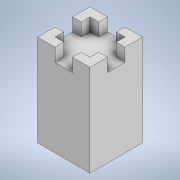
# Autodesk Inventor part: rook
Saved by Autodesk Inventor 2021 (Build 250183000, 183)
## iProperties
Created: 2021-01-20
Part Number: rook
Material: Generic
Document SubType Name: Modeling
Designer: Luke Kamols
Density: 1 g/cm^3
Appearance: Default
Author: Luke Kamols
Autodesk Inventor part; units mm, degrees
ref_plane "YZ Plane" through (0, 0, 0) normal (1, 0, 0) x (0, 1, 0)
ref_plane "XZ Plane" through (0, 0, 0) normal (0, 1, 0) x (-1, 0, 0)
ref_plane "XY Plane" through (0, 0, 0) normal (0, 0, 1) x (1, 0, 0)
sketch "Sketch1" plane through (0, 0, 0) normal (0, 1, 0) x (-1, 0, 0)
  line L0 (0, 0) -> (20, 0)
  line L1 (20, 0) -> (20, -20)
  line L2 (20, -20) -> (0, -20)
  line L3 (0, -20) -> (0, 0)
  dimension "d0" = 20
  dimension "d1" = 20
  constraints: 8 end point, 2 parallel, 1 horizontal, 1 perpendicular
  measures "d0" distance of L1.end L2.end
  measures "d1" distance of L0.end L1.end
extrude "Extrusion1" add sketch "Sketch1" along normal blind 30
sketch "Sketch2" plane through (0, 30, 0) normal (0, 1, 0) x (1, 0, 0)
  line L0 (0, 20) -> (-20, 20) projected
  line L1 (-20, 20) -> (-20, 0) projected
  line L2 (-20, 0) -> (0, 0) projected
  line L3 (0, 0) -> (0, 20) projected
  line L4 (0, 0) -> (0, 20) projected
  line L5 (0, 0) -> (0, 6.66)
  line L6 (0, 6.66) -> (-3.33, 6.66)
  line L7 (-3.33, 6.66) -> (-3.33, 3.33)
  line L8 (-3.33, 3.33) -> (-6.66, 3.33)
  line L9 (-6.66, 3.33) -> (-6.66, 0)
  line L10 (-20, 0) -> (0, 0) projected
  line L11 (-10, 0) -> (-10, 20)
  line L12 (0, 20) -> (-20, 20) projected
  line L13 (0, 10) -> (-20, 10)
  line L14 (-20, 20) -> (-20, 0) projected
  line L15 (-20, 6.66) -> (-16.67, 6.66)
  line L16 (-16.67, 6.66) -> (-16.67, 3.33)
  line L17 (-16.67, 3.33) -> (-13.34, 3.33)
  line L18 (-13.34, 3.33) -> (-13.34, 0)
  line L19 (0, 13.34) -> (-3.33, 13.34)
  line L20 (-3.33, 13.34) -> (-3.33, 16.67)
  line L21 (-3.33, 16.67) -> (-6.66, 16.67)
  line L22 (-6.66, 16.67) -> (-6.66, 20)
  line L23 (-20, 13.34) -> (-16.67, 13.34)
  line L24 (-16.67, 13.34) -> (-16.67, 16.67)
  line L25 (-16.67, 16.67) -> (-13.34, 16.67)
  line L26 (-13.34, 16.67) -> (-13.34, 20)
  point P0 (-6.66, 20)
  point P1 (-13.34, 20)
  point P2 (-20, 6.66)
  point P3 (-13.34, 0)
  dimension "d4" = 6.66
  dimension "d5" = 3.33
  dimension "d6" = 3.33
  dimension "d7" = 3.33
  constraints: 38 end point, 15 symmetric about line, 4 midpoint, 4 perpendicular, 2 point on line
  measures "d4" distance of L4.start L5.end
  measures "d5" distance of L5.end L6.end
  measures "d6" distance of L6.end L7.end
  measures "d7" distance of L7.end L8.end
extrude "Extrusion2" add sketch "Sketch2" along normal blind 5 contours L3 L19 L20 L21 L22 L0 | L26 L25 L24 L23 L1 L0 | L3 L2 L9 L8 L7 L6 | L2 L1 L15 L16 L17 L18
body "Solid1"
